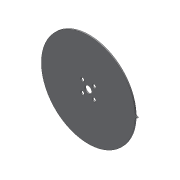
# Autodesk Inventor part: IndPlate
Saved by Autodesk Inventor 2018 (Build 220112000, 112)
## iProperties
Created: 2019-09-26
Part Number: IndPlate
Material: Generic
Document SubType Name: Modeling
Designer: Clevo
Density: 1 g/cm^3
Appearance: Default
Author: Clevo
Autodesk Inventor part; units mm, degrees
ref_plane "YZ Plane" through (0, 0, 0) normal (1, 0, 0) x (0, 1, 0)
ref_plane "XZ Plane" through (0, 0, 0) normal (0, 1, 0) x (-1, 0, 0)
ref_plane "XY Plane" through (0, 0, 0) normal (0, 0, 1) x (1, 0, 0)
sketch "Sketch1" plane through (0, 0, 0) normal (0, 1, 0) x (-1, 0, 0)
  circle A0 centre (0, 0) radius 40
  dimension "d2" = 80
  constraints: 1 centre point, 1 coincident
  measures "d2" diameter of A0
extrude "Extrusion1" add sketch "Sketch1" along normal blind 1
sketch "Sketch2" plane through (0, 1, 0) normal (0, 1, 0) x (1, 0, 0)
  circle A0 centre (0, 0) radius 3
  dimension "d3" = 6
  constraints: 1 centre point, 1 coincident
  measures "d3" diameter of A0
extrude "Extrusion2" cut sketch "Sketch2" against normal through all
sketch "Sketch3" plane through (0, 1, 0) normal (0, 1, 0) x (1, 0, 0)
  line L0 (4.9497, 4.9497) -> (-4.9497, 4.9497)
  line L1 (-4.9497, 4.9497) -> (-4.9497, -4.9497)
  line L2 (-4.9497, -4.9497) -> (4.9497, -4.9497)
  line L3 (4.9497, -4.9497) -> (4.9497, 4.9497)
  circle A0 centre (0, 0) radius 3 projected
  line L4 (4.9497, 4.9497) -> (-4.9497, -4.9497) construction
  line L5 (-4.9497, 4.9497) -> (4.9497, -4.9497) construction
  dimension "d6" = 14
  dimension "d7" = 14
  dimension "d8" = 9.8995
  dimension "d9" = 9.8995
  constraints: 12 end point, 2 midpoint, 2 parallel, 1 horizontal, 1 perpendicular
  measures "d6" distance of L0.end L2.end
  measures "d7" distance of L0.start L1.end
  measures "d8" distance of L0.end L1.end
  measures "d9" distance of L1.end L2.end
hole "Hole1" at (-4.9497, 1, 4.9497) at (-4.9497, 1, -4.9497) at (4.9497, 1, 4.9497) at (4.9497, 1, -4.9497) direction (0, -1, 0) diameter 3.2 end through all clearance for "Flat Head Machine Screw" size "M3" standard "Ansi Metric M Profile"
sketch "Sketch4" plane through (0, 0, 0) normal (0, -1, 0) x (1, 0, 0)
  circle A0 centre (4.9497, 4.9497) radius 1.6 projected
  circle A1 centre (-4.9497, 4.9497) radius 1.6 projected
  circle A2 centre (-4.9497, -4.9497) radius 1.6 projected
  circle A3 centre (4.9497, -4.9497) radius 1.6 projected
  circle A4 centre (0, 0) radius 3 projected
  circle A5 centre (0, 0) radius 40 projected
  circle A6 centre (0, 0) radius 40 projected
  line L0 (39.9875, 1) -> (42, 0)
  line L1 (42, 0) -> (39.9875, -1)
  dimension "d18" = 1
  dimension "d19" = 1
  dimension "d20" = 42
  constraints: 4 end point, 2 point on circle, 1 horizontal alignment
  measures "d18" vertical distance of L0.end L0.start
  measures "d19" vertical distance of L0.end L1.end
  measures "d20" distance of point (0, 0) L0.end
extrude "Extrusion3" add sketch "Sketch4" against normal blind 1 contours A5 L0 L1
fillet "Fillet1" radius 1 2 edges at (39.9875, 0.5, -1) (39.9875, 0.5, 1)
equation "\"d8\" = d9"
equation "\"d19\" = d18"
body "Solid1"
